Autodesk Fusion 360 part; units mm, degrees
(part 2 of 2)
sketch "Esquisse13" plane through (0, -12, 0) normal (0, -1, 0) x (1, 0, 0)
  line L0 (-488.8, 12) -> (-363.6, 12)
  line L1 (-363.6, 12) -> (-363.6, 0)
  line L2 (-363.6, 0) -> (-488.8, 0)
  line L3 (-488.8, 0) -> (-488.8, 12)
  line L4 (-238.4, 0) -> (-238.4, 12)
  line L5 (-238.4, 12) -> (-113.2, 12)
  line L6 (-113.2, 12) -> (-113.2, 0)
  line L7 (-113.2, 0) -> (-238.4, 0)
  circle A0 centre (-508.8, 6) radius 2
  circle A1 centre (-343.6, -186) radius 2
  circle A2 centre (-8, -186) radius 2
  circle A3 centre (-93.2, -186) radius 2
  circle A4 centre (-258.4, 6) radius 2
  circle A5 centre (-594, -186) radius 2
  circle A6 centre (-594, 6) radius 2
  circle A7 centre (-8, 6) radius 2
  circle A8 centre (-258.4, -186) radius 2
  circle A9 centre (-93.2, 6) radius 2
  circle A10 centre (-343.6, 6) radius 2
  circle A11 centre (-508.8, -186) radius 2
  line L8 (-363.6, -180) -> (-363.6, -192)
  line L9 (-363.6, -192) -> (-488.8, -192)
  line L10 (-488.8, -192) -> (-488.8, -180)
  line L11 (-488.8, -180) -> (-363.6, -180)
  line L12 (-238.4, -180) -> (-113.2, -180)
  line L13 (-113.2, -180) -> (-113.2, -192)
  line L14 (-113.2, -192) -> (-238.4, -192)
  line L15 (-238.4, -192) -> (-238.4, -180)
  line L16 (0, -332) -> (12, -332)
  line L17 (12, -332) -> (12, -241)
  line L18 (12, -241) -> (0, -241)
  line L19 (0, -241) -> (0, -150)
  line L20 (0, -150) -> (12, -150)
  line L21 (12, -150) -> (12, -59)
  line L22 (12, -59) -> (0, -59)
  line L23 (0, -59) -> (0, 32)
  line L24 (0, 32) -> (-602, 32)
  line L25 (-602, 32) -> (-602, -59)
  line L26 (-602, -59) -> (-614, -59)
  line L27 (-614, -59) -> (-614, -150)
  line L28 (-614, -150) -> (-602, -150)
  line L29 (-602, -150) -> (-602, -241)
  line L30 (-602, -241) -> (-614, -241)
  line L31 (-614, -241) -> (-614, -332)
  line L32 (-614, -332) -> (-602, -332)
  line L33 (-602, -332) -> (-602, -423)
  line L34 (-602, -423) -> (-614, -423)
  line L35 (-614, -423) -> (-614, -514)
  line L36 (-614, -514) -> (-602, -514)
  line L37 (-602, -514) -> (-602, -593)
  line L38 (-602, -593) -> (0, -593)
  line L39 (0, -593) -> (0, -514)
  line L40 (0, -514) -> (12, -514)
  line L41 (12, -514) -> (12, -423)
  line L42 (12, -423) -> (0, -423)
  line L43 (0, -423) -> (0, -332)
  line L44 (-602, 32) -> (0, 32)
  line L45 (0, 32) -> (0, -593)
  line L46 (0, -593) -> (-602, -593)
  line L47 (-602, -593) -> (-602, 32)
  line L48 (-20, -573) -> (-582, -573)
  line L49 (-582, -573) -> (-582, 12)
  line L50 (-582, 12) -> (-20, 12)
  line L51 (-20, 12) -> (-20, -573)
  line L52 (-582, -270.5) -> (-20, -270.5)
  line L53 (-20, -270.5) -> (-20, -290.5)
  line L54 (-20, -290.5) -> (-582, -290.5)
  line L55 (-582, -290.5) -> (-582, -270.5)
  dimension "d175" = 20
  dimension "d176" = 20
  constraint horizontal L44
  constraint vertical L45
  constraint horizontal L46
  constraint vertical L47
  constraint coincident L38.end L39.start
  constraint coincident L24.end L25.start
  constraint horizontal L52
  constraint vertical L53
  constraint horizontal L54
  constraint vertical L55
  constraint midpoint L51 L53
  constraint midpoint L49 L55
  measures "d176" distance of L52.end L53.end
extrude "Extrusion15" add sketch "Esquisse13" along normal blind 20 separate body contours L49 L51 L52 L53 L54 L55 | L19 L23 L24 L25 L29 L33 L37 L38 L39 L43 L44 L45 L46 L47 makes body 7
extrude "Extrusion16" cut sketch "Esquisse4" along normal blind 12 contours A12 L58 L76 | A12 L58 | A12 L76 bodies 3
sketch "Esquisse15" plane through (0, 0, 12) normal (0, 0, 1) x (1, 0, 0)
  line L0 (0, 845.1428) -> (0, 988)
  line L1 (0, 988) -> (-602, 988)
  line L2 (-602, 988) -> (-602, 845.1428)
  line L3 (-602, 845.1428) -> (-614, 845.1428)
  line L4 (-614, 845.1428) -> (-614, 702.2857)
  line L5 (-614, 702.2857) -> (-602, 702.2857)
  line L6 (-602, 702.2857) -> (-602, 559.4286)
  line L7 (-602, 559.4286) -> (-614, 559.4286)
  line L8 (-614, 559.4286) -> (-614, 416.5714)
  line L9 (-614, 416.5714) -> (-602, 416.5714)
  line L10 (-602, 416.5714) -> (-602, 273.7143)
  line L11 (-602, 273.7143) -> (-614, 273.7143)
  line L12 (-614, 273.7143) -> (-614, 130.8571)
  line L13 (-614, 130.8571) -> (-602, 130.8571)
  line L14 (-602, 130.8571) -> (-602, 0)
  line L15 (-602, 0) -> (-488.8, 0)
  line L16 (-488.8, 0) -> (-488.8, -12)
  line L17 (-488.8, -12) -> (-363.6, -12)
  line L18 (-363.6, -12) -> (-363.6, 0)
  line L19 (-363.6, 0) -> (-238.4, 0)
  line L20 (-238.4, 0) -> (-238.4, -12)
  line L21 (-238.4, -12) -> (-113.2, -12)
  line L22 (-113.2, -12) -> (-113.2, 0)
  line L23 (-113.2, 0) -> (0, 0)
  line L24 (0, 0) -> (0, 130.8571)
  line L25 (0, 130.8571) -> (12, 130.8571)
  line L26 (12, 130.8571) -> (12, 273.7143)
  line L27 (12, 273.7143) -> (0, 273.7143)
  line L28 (0, 273.7143) -> (0, 416.5714)
  line L29 (0, 416.5714) -> (12, 416.5714)
  line L30 (12, 416.5714) -> (12, 559.4286)
  line L31 (12, 559.4286) -> (0, 559.4286)
  line L32 (0, 559.4286) -> (0, 702.2857)
  line L33 (0, 702.2857) -> (12, 702.2857)
  line L34 (12, 702.2857) -> (12, 845.1428)
  line L35 (12, 845.1428) -> (0, 845.1428)
  line L36 (-301, 0) -> (-301, 988) construction
  circle A0 centre (-301, 40) radius 4
  circle A1 centre (-301, 390) radius 4
  circle A2 centre (-301, 740) radius 4
  dimension "d263" = 8
  dimension "d264" = 40
  dimension "d267" = 0
  dimension "d268" = 350
  constraint midpoint L19 L36.start
  constraint midpoint L1 L36.end
  constraint coincident L36 A0.centre
  measures "d263" diameter of A0
  measures "d264" distance of L36.start A0.centre
extrude "Extrusion17" cut sketch "Esquisse15" against normal blind 12 contours A0 | A1 | A2 bodies 5
copy_body "Corps->Comp1" bodies 1 removing the originals makes body 8 in component "Component"
copy_body "Corps->Comp2" bodies 6 removing the originals makes body 9 in component "Component'"
copy_body "Corps->Comp3" bodies 2 removing the originals makes body 10 in component "Component''"
copy_body "Corps->Comp4" bodies 4 removing the originals makes body 11 in component "Component'''"
copy_body "Corps->Comp5" bodies 5 removing the originals makes body 12 in component "Component''''"
copy_body "Corps->Comp6" bodies 3 removing the originals makes body 13 in component "Component'''''"
copy_body "Corps->Comp7" bodies 7 removing the originals makes body 14 in component "Component''''''"
sketch "Esquisse14" plane through (0, 0, 0) normal (0, 1, 0) x (1, 0, 0)
  line L0 (0, 0) -> (1250, 0)
  line L1 (1250, 0) -> (1250, -4000)
  line L2 (1250, -4000) -> (0, -4000)
  line L3 (0, -4000) -> (0, 0)
  line L4 (0, -4000) -> (-1250, -4000)
  line L5 (-1250, -4000) -> (-1250, 0)
  line L6 (-1250, 0) -> (0, 0)
  line L7 (0, 0) -> (0, -4000)
  line L8 (-1250, -4000) -> (-1650, -4000)
  line L9 (-1650, -4000) -> (-1650, 0)
  line L10 (-1650, 0) -> (-1250, 0)
  line L11 (-1250, 0) -> (-1250, -4000)
  dimension "d179" = 1250
  dimension "d180" = 4000
  dimension "d192" = 1250
  dimension "d193" = 400
  constraint horizontal L0
  constraint vertical L1
  constraint horizontal L2
  constraint vertical L3
  constraint coincident L0.start L3.end
  constraint horizontal L4
  constraint vertical L5
  constraint horizontal L6
  constraint vertical L7
  constraint horizontal L8
  constraint vertical L9
  constraint horizontal L10
  constraint vertical L11
  measures "d179" distance of L0.start L0.end
  measures "d180" distance of L0.start L2.end
  measures "d192" distance of L2.end L4.end
  measures "d193" distance of L9.end L5.end
other "Réorganiser1"
sketch "Esquisse1 (2)" plane through (0, 0, 0) normal (0, 1, 0) x (0, 0, -1) in component "Component'''''"
  circle A0 centre (-6, 508.8) radius 2
  circle A1 centre (186, 343.6) radius 2
  circle A2 centre (186, 8) radius 2
  circle A3 centre (186, 93.2) radius 2
  circle A4 centre (-6, 258.4) radius 2
  circle A5 centre (186, 594) radius 2
  circle A6 centre (-6, 594) radius 2
  circle A7 centre (-6, 8) radius 2
  circle A8 centre (186, 258.4) radius 2
  circle A9 centre (-6, 93.2) radius 2
  circle A10 centre (-6, 343.6) radius 2
  circle A11 centre (186, 508.8) radius 2
  line L0 (59, 602) -> (-32, 602)
  line L1 (-32, 290.802) -> (-32, 0)
  line L2 (-32, 0) -> (59, 0)
  line L3 (59, 0) -> (59, -12)
  line L4 (59, -12) -> (150, -12)
  line L5 (150, -12) -> (150, 0)
  line L6 (150, 0) -> (241, 0)
  line L7 (241, 0) -> (241, -12)
  line L8 (241, -12) -> (332, -12)
  line L9 (332, -12) -> (332, 0)
  line L10 (332, 0) -> (423, 0)
  line L11 (423, 0) -> (423, -12)
  line L12 (423, -12) -> (514, -12)
  line L13 (514, -12) -> (514, 0)
  line L14 (514, 0) -> (593, 0)
  line L15 (593, 0) -> (593, 602)
  line L16 (593, 602) -> (514, 602)
  line L17 (514, 602) -> (514, 614)
  line L18 (514, 614) -> (423, 614)
  line L19 (423, 614) -> (423, 602)
  line L20 (423, 602) -> (332, 602)
  line L21 (332, 602) -> (332, 614)
  line L22 (332, 614) -> (241, 614)
  line L23 (241, 614) -> (241, 602)
  line L24 (241, 602) -> (150, 602)
  line L25 (150, 602) -> (150, 614)
  line L26 (150, 614) -> (59, 614)
  line L27 (59, 614) -> (59, 602)
  line L28 (-12, 488.8) -> (0, 488.8)
  line L29 (0, 488.8) -> (0, 363.6)
  line L30 (0, 363.6) -> (-12, 363.6)
  line L31 (-12, 363.6) -> (-12, 488.8)
  line L32 (180, 488.8) -> (192, 488.8)
  line L33 (192, 488.8) -> (192, 363.6)
  line L34 (192, 363.6) -> (180, 363.6)
  line L35 (180, 363.6) -> (180, 488.8)
  line L36 (180, 238.4) -> (192, 238.4)
  line L37 (192, 238.4) -> (192, 113.2)
  line L38 (192, 113.2) -> (180, 113.2)
  line L39 (180, 113.2) -> (180, 238.4)
  line L40 (-12, 238.4) -> (0, 238.4)
  line L41 (0, 238.4) -> (0, 113.2)
  line L42 (0, 113.2) -> (-12, 113.2)
  line L43 (-12, 113.2) -> (-12, 238.4)
  arc A12 (-32, 290.802) -> (-32, 311.198) centre (-24.6, 301) ccw
  line L44 (-32, 602) -> (-32, 311.198)
  point P0 (-9.6665, 115.5335)
  point P1 (-9.6665, 236.0665)
  point P2 (-2.3335, 236.0665)
  point P3 (-2.3335, 115.5335)
  point P4 (-2.3335, 486.4665)
  point P5 (-2.3335, 365.9335)
  point P6 (-9.6665, 486.4665)
  point P7 (-9.6665, 365.9335)
  point P8 (182.3335, 115.5335)
  point P9 (182.3335, 236.0665)
  point P10 (189.6665, 236.0665)
  point P11 (189.6665, 115.5335)
  point P12 (189.6665, 486.4665)
  point P13 (189.6665, 365.9335)
  point P14 (182.3335, 486.4665)
  point P15 (182.3335, 365.9335)
  point P16 (56.6665, 604.3335)
  point P17 (152.3335, 604.3335)
  point P18 (238.6665, 604.3335)
  point P19 (334.3335, 604.3335)
  point P20 (420.6665, 604.3335)
  point P21 (516.3335, 604.3335)
  point P22 (56.6665, -2.3335)
  point P23 (152.3335, -2.3335)
  point P24 (238.6665, -2.3335)
  point P25 (334.3335, -2.3335)
  point P26 (420.6665, -2.3335)
  point P27 (516.3335, -2.3335)
hole "Perçage1" at (-115.5335, 0, 9.6665) at (-236.0665, 0, 9.6665) at (-236.0665, 0, 2.3335) at (-115.5335, 0, 2.3335) at (-486.4665, 0, 2.3335) at (-365.9335, 0, 2.3335) at (-486.4665, 0, 9.6665) at (-365.9335, 0, 9.6665) at (-115.5335, 0, -182.3335) at (-236.0665, 0, -182.3335) at (-236.0665, 0, -189.6665) at (-115.5335, 0, -189.6665) at (-486.4665, 0, -189.6665) at (-365.9335, 0, -189.6665) at (-486.4665, 0, -182.3335) at (-365.9335, 0, -182.3335) direction (0, -1, 0) diameter 6 depth 12 tip angle 180 bodies 13 in component "Component'''''"
hole "Perçage2" at (-604.3335, 0, -56.6665) at (-604.3335, 0, -152.3335) at (-604.3335, 0, -238.6665) at (-604.3335, 0, -334.3335) at (-604.3335, 0, -420.6665) at (-604.3335, 0, -516.3335) at (2.3335, 0, -56.6665) at (2.3335, 0, -152.3335) at (2.3335, 0, -238.6665) at (2.3335, 0, -334.3335) at (2.3335, 0, -420.6665) at (2.3335, 0, -516.3335) direction (0, -1, 0) diameter 6 depth 12 tip angle 180 bodies 13 in component "Component'''''"
sketch "Esquisse1 (3)" plane through (0, 0, -605) normal (0, 0, -1) x (-1, 0, 0) in component "Component'"
  spline S0 degree 3 poles (527.6621, 131.6413) (528.5608, 136.7718) (530.453, 141.6777) (536.0113, 150.4881) (539.6243, 154.3083) (547.2342, 159.7245) (550.9515, 161.5844) (558.8233, 164.0997) (562.9304, 164.7399) (567.0623, 164.7399) knots 0 0 0 0 1.562578 1.562578 3.125156 3.125156 4.364729 4.364729 5.604303 5.604303 5.604303 5.604303
  spline S1 degree 5 poles (527.6621, 131.6413) (526.9913, 127.8114) (525.3201, 119.0874) (522.2246, 106.0357) (516.6629, 89.886) (506.2841, 73.0853) (490.6132, 60.2852) (469.9401, 52.3455) (445.0295, 48.3011) (417.063, 46.7974) (393.2682, 46.4893) (375.0825, 46.2548) (362.8686, 46.0302) (356.739, 45.9008) knots 0.124254 0.124254 0.124254 0.124254 0.124254 0.124254 0.2 0.3 0.4 0.5 0.6 0.7 0.8 0.9 1 1 1 1 1 1
  line L0 (356.739, 45.9008) -> (245.261, 45.9008)
  spline S2 degree 5 poles (245.261, 45.9008) (239.1314, 46.0302) (226.9175, 46.2548) (208.7318, 46.4893) (184.937, 46.7974) (156.9705, 48.3011) (132.0599, 52.3455) (111.3868, 60.2852) (95.7159, 73.0853) (85.3371, 89.886) (79.7754, 106.0357) (76.6799, 119.0874) (75.0087, 127.8114) (74.3379, 131.6413) knots -1 -1 -1 -1 -1 -1 -0.9 -0.8 -0.7 -0.6 -0.5 -0.4 -0.3 -0.2 -0.124254 -0.124254 -0.124254 -0.124254 -0.124254 -0.124254
  spline S3 degree 3 poles (34.9377, 164.7399) (40.1463, 164.7399) (45.3051, 163.7226) (54.9424, 159.7677) (59.3287, 156.8679) (65.9766, 150.3067) (68.45, 146.966) (72.2857, 139.6463) (73.625, 135.7113) (74.3379, 131.6413) knots 0 0 0 0 1.562578 1.562578 3.125156 3.125156 4.364729 4.364729 5.604303 5.604303 5.604303 5.604303
  line L1 (34.9377, 164.7399) -> (-6, 164.7399)
  line L2 (-6, 164.7399) -> (-6, 158.7399)
  line L3 (-6, 158.7399) -> (0, 158.7399)
  line L4 (0, 158.7399) -> (0, -44.13)
  line L5 (0, -44.13) -> (-12, -44.13)
  line L6 (-12, -44.13) -> (-12, -56.13)
  line L7 (-12, -56.13) -> (614, -56.13)
  line L8 (614, -56.13) -> (614, -44.13)
  line L9 (614, -44.13) -> (602, -44.13)
  line L10 (602, -44.13) -> (602, 158.7399)
  line L11 (602, 158.7399) -> (608, 158.7399)
  line L12 (608, 158.7399) -> (608, 164.7399)
  line L13 (608, 164.7399) -> (567.0623, 164.7399)
  point P0 (604.3335, 156.4065)
  point P1 (-2.3335, 156.4065)
  point P2 (-2.3335, -41.7966)
  point P3 (604.3335, -41.7966)
hole "Perçage1'" at (-604.3335, 156.4065, -605) at (2.3335, 156.4065, -605) direction (0, 0, 1) diameter 6 depth 6 tip angle 180 bodies 9 in component "Component'"
hole "Perçage2'" at (2.3335, -41.7966, -605) at (-604.3335, -41.7966, -605) direction (0, 0, 1) diameter 6 depth 12 tip angle 180 bodies 9 in component "Component'"
sketch "Esquisse1 (4)" plane through (0, 0, 12) normal (0, 0, 1) x (0, 1, 0) in component "Component''''"
  line L0 (845.1428, 0) -> (988, 0)
  line L1 (988, 0) -> (988, 602)
  line L2 (988, 602) -> (845.1428, 602)
  line L3 (845.1428, 602) -> (845.1428, 614)
  line L4 (845.1428, 614) -> (702.2857, 614)
  line L5 (702.2857, 614) -> (702.2857, 602)
  line L6 (702.2857, 602) -> (559.4286, 602)
  line L7 (559.4286, 602) -> (559.4286, 614)
  line L8 (559.4286, 614) -> (416.5714, 614)
  line L9 (416.5714, 614) -> (416.5714, 602)
  line L10 (416.5714, 602) -> (273.7143, 602)
  line L11 (273.7143, 602) -> (273.7143, 614)
  line L12 (273.7143, 614) -> (130.8571, 614)
  line L13 (130.8571, 614) -> (130.8571, 602)
  line L14 (130.8571, 602) -> (0, 602)
  line L15 (0, 602) -> (0, 488.8)
  line L16 (0, 488.8) -> (-12, 488.8)
  line L17 (-12, 488.8) -> (-12, 363.6)
  line L18 (-12, 363.6) -> (0, 363.6)
  line L19 (0, 363.6) -> (0, 238.4)
  line L20 (0, 238.4) -> (-12, 238.4)
  line L21 (-12, 238.4) -> (-12, 113.2)
  line L22 (-12, 113.2) -> (0, 113.2)
  line L23 (0, 113.2) -> (0, 0)
  line L24 (0, 0) -> (130.8571, 0)
  line L25 (130.8571, 0) -> (130.8571, -12)
  line L26 (130.8571, -12) -> (273.7143, -12)
  line L27 (273.7143, -12) -> (273.7143, 0)
  line L28 (273.7143, 0) -> (416.5714, 0)
  line L29 (416.5714, 0) -> (416.5714, -12)
  line L30 (416.5714, -12) -> (559.4286, -12)
  line L31 (559.4286, -12) -> (559.4286, 0)
  line L32 (559.4286, 0) -> (702.2857, 0)
  line L33 (702.2857, 0) -> (702.2857, -12)
  line L34 (702.2857, -12) -> (845.1428, -12)
  line L35 (845.1428, -12) -> (845.1428, 0)
  circle A0 centre (40, 301) radius 4
  circle A1 centre (390, 301) radius 4
  circle A2 centre (740, 301) radius 4
  point P0 (-2.3335, 491.1335)
  point P1 (-2.3335, 361.2665)
  point P2 (-2.3335, 240.7335)
  point P3 (-2.3335, 110.8665)
  point P4 (128.5237, 604.3335)
  point P5 (276.0477, 604.3335)
  point P6 (414.238, 604.3335)
  point P7 (699.9523, 604.3335)
  point P8 (847.4763, 604.3335)
  point P9 (561.762, 604.3335)
  point P10 (414.238, -2.3335)
  point P11 (561.762, -2.3335)
  point P12 (276.0477, -2.3335)
  point P13 (699.9523, -2.3335)
  point P14 (128.5237, -2.3335)
  point P15 (847.4763, -2.3335)
hole "Perçage1''" at (-491.1335, -2.3335, 12) at (-361.2665, -2.3335, 12) at (-240.7335, -2.3335, 12) at (-110.8665, -2.3335, 12) direction (0, 0, -1) diameter 6 depth 12 tip angle 180 bodies 12 in component "Component''''"
hole "Perçage2''" at (-604.3335, 276.0477, 12) at (-604.3335, 414.238, 12) at (-604.3335, 699.9523, 12) at (-604.3335, 847.4763, 12) at (-604.3335, 561.762, 12) at (2.3335, 414.238, 12) at (2.3335, 561.762, 12) at (2.3335, 276.0477, 12) at (2.3335, 699.9523, 12) at (2.3335, 128.5237, 12) at (2.3335, 847.4763, 12) direction (0, 0, -1) diameter 6 depth 12 tip angle 180 bodies 12 in component "Component''''"
hole "Perçage3" at (-604.3335, 128.5237, 12) direction (0, 0, -1) diameter 6 depth 12 tip angle 180 bodies 12 in component "Component''''"
sketch "Esquisse1 (5)" plane through (0, 0, 0) normal (-1, 0, 0) x (0, 0, 1) in component "Component"
  arc A0 (32.1287, 968) -> (12.1287, 988) centre (12.1287, 968) ccw
  line L0 (12.1287, 988) -> (-209.8465, 988)
  arc A1 (-209.8465, 988) -> (-227.5983, 977.2127) centre (-209.8465, 968) ccw
  line L1 (-227.5983, 977.2127) -> (-569.8721, 317.6877)
  arc A2 (-569.8721, 317.6877) -> (-605, 173.7399) centre (-292.5, 173.7399) ccw
  line L2 (-605, 173.7399) -> (-593, 173.7399)
  line L3 (-593, 173.7399) -> (-593, 158.7399)
  line L4 (-593, 158.7399) -> (-593, 150.7399)
  line L5 (-593, 150.7399) -> (-599, 150.7399)
  line L6 (-599, 150.7399) -> (-599, 158.7399)
  line L7 (-599, 158.7399) -> (-605, 158.7399)
  line L8 (-605, 158.7399) -> (-605, 16.37)
  line L9 (-605, 16.37) -> (-626.1765, -28.9242)
  arc A3 (-626.1765, -28.9242) -> (-585.3674, -68.3537) centre (-599, -41.63) ccw
  line L10 (-585.3674, -68.3537) -> (-514.1044, -32)
  line L11 (-514.1044, -32) -> (12, -32)
  arc A4 (12, -32) -> (32, -12) centre (12, -12) ccw
  line L12 (32, -12) -> (32.1287, -12)
  line L13 (32.1287, -12) -> (32.1287, 968)
  line L14 (-59, 0) -> (-59, -12)
  line L15 (-59, -12) -> (-150, -12)
  line L16 (-150, -12) -> (-150, 0)
  line L17 (-150, 0) -> (-59, 0)
  line L18 (-192, 273.7143) -> (-180, 273.7143)
  line L19 (-180, 273.7143) -> (-180, 130.8571)
  line L20 (-180, 130.8571) -> (-192, 130.8571)
  line L21 (-192, 130.8571) -> (-192, 273.7143)
  line L22 (-180, 559.4286) -> (-180, 416.5714)
  line L23 (-180, 416.5714) -> (-192, 416.5714)
  line L24 (-192, 416.5714) -> (-192, 559.4286)
  line L25 (-192, 559.4286) -> (-180, 559.4286)
  line L26 (0, 702.2857) -> (0, 845.1428)
  line L27 (0, 845.1428) -> (12, 845.1428)
  line L28 (12, 845.1428) -> (12, 702.2857)
  line L29 (12, 702.2857) -> (0, 702.2857)
  line L30 (-241, 0) -> (-241, -12)
  line L31 (-241, -12) -> (-332, -12)
  line L32 (-332, -12) -> (-332, 0)
  line L33 (-332, 0) -> (-241, 0)
  line L34 (0, 130.8571) -> (0, 273.7143)
  line L35 (0, 273.7143) -> (12, 273.7143)
  line L36 (12, 273.7143) -> (12, 130.8571)
  line L37 (12, 130.8571) -> (0, 130.8571)
  line L38 (-180, 845.1428) -> (-180, 702.2857)
  line L39 (-180, 702.2857) -> (-192, 702.2857)
  line L40 (-192, 702.2857) -> (-192, 845.1428)
  line L41 (-192, 845.1428) -> (-180, 845.1428)
  line L42 (0, 416.5714) -> (0, 559.4286)
  line L43 (0, 559.4286) -> (12, 559.4286)
  line L44 (12, 559.4286) -> (12, 416.5714)
  line L45 (12, 416.5714) -> (0, 416.5714)
  line L46 (-423, 0) -> (-423, -12)
  line L47 (-423, -12) -> (-514, -12)
  line L48 (-514, -12) -> (-514, 0)
  line L49 (-514, 0) -> (-423, 0)
  line L50 (-593, -27.13) -> (-593, -35.13)
  arc A5 (-593, -48.13) -> (-593, -35.13) centre (-599, -41.63) ccw
  line L51 (-593, -48.13) -> (-593, -56.13)
  line L52 (-593, -56.13) -> (-605, -56.13)
  line L53 (-605, -56.13) -> (-605, -48.13)
  arc A6 (-605, -35.13) -> (-605, -48.13) centre (-599, -41.63) ccw
  line L54 (-605, -35.13) -> (-605, -27.13)
  line L55 (-605, -27.13) -> (-593, -27.13)
  circle A7 centre (6, 115.8571) radius 2
  circle A8 centre (-161.8713, -6) radius 2
  circle A9 centre (6, 288.7143) radius 2
  circle A10 centre (6, 401.5714) radius 2
  circle A11 centre (-229, -6) radius 2
  circle A12 centre (-343.8713, -6) radius 2
  circle A13 centre (6, 574.4286) radius 2
  circle A14 centre (6, 687.2857) radius 2
  circle A15 centre (6, 860.1428) radius 2
  circle A16 centre (-525.8713, -6) radius 2
  circle A17 centre (-581, -6) radius 2
  circle A18 centre (-186, 687.2857) radius 2
  circle A19 centre (-411, -6) radius 2
  circle A20 centre (6, 15) radius 2
  circle A21 centre (6, 973) radius 2
  circle A22 centre (-186, 288.7143) radius 2
  circle A23 centre (-186, 860.1428) radius 2
  circle A24 centre (-186, 973) radius 2
  circle A25 centre (-186, 401.5714) radius 2
  circle A26 centre (-186, 574.4286) radius 2
  circle A27 centre (-186, 15) radius 2
  circle A28 centre (-186, 115.8571) radius 2
  circle A29 centre (20.1287, -6) radius 2
  circle A30 centre (-47, -6) radius 2
  point P0 (-61.3335, -2.3335)
  point P1 (-61.3335, -9.6665)
  point P2 (-147.6665, -2.3335)
  point P3 (-147.6665, -9.6665)
  point P4 (-189.6665, 271.3808)
  point P5 (-182.3335, 271.3808)
  point P6 (-189.6665, 133.1906)
  point P7 (-182.3335, 133.1906)
  point P8 (-182.3335, 557.0951)
  point P9 (-182.3335, 418.9049)
  point P10 (-189.6665, 557.0951)
  point P11 (-189.6665, 418.9049)
  point P12 (2.3335, 704.6192)
  point P13 (2.3335, 842.8094)
  point P14 (9.6665, 704.6192)
  point P15 (9.6665, 842.8094)
  point P16 (-243.3335, -2.3335)
  point P17 (-243.3335, -9.6665)
  point P18 (-329.6665, -2.3335)
  point P19 (-329.6665, -9.6665)
  point P20 (2.3335, 133.1906)
  point P21 (2.3335, 271.3808)
  point P22 (9.6665, 133.1906)
  point P23 (9.6665, 271.3808)
  point P24 (-182.3335, 842.8094)
  point P25 (-182.3335, 704.6192)
  point P26 (-189.6665, 842.8094)
  point P27 (-189.6665, 704.6192)
  point P28 (2.3335, 418.9049)
  point P29 (2.3335, 557.0951)
  point P30 (9.6665, 418.9049)
  point P31 (9.6665, 557.0951)
  point P32 (-425.3335, -2.3335)
  point P33 (-425.3335, -9.6665)
  point P34 (-511.6665, -2.3335)
  point P35 (-511.6665, -9.6665)
  point P36 (-595.3335, -29.4635)
  point P37 (-602.6665, -29.4635)
  point P38 (-595.3335, -53.7966)
  point P39 (-602.6665, -53.7966)
  point P40 (-608.2214, 17.0858)
  point P41 (-513.3333, -35.2086)
  point P42 (-595.3335, 153.0734)
  point P43 (-596.6665, 153.0734)
  point P44 (-595.3335, 171.4065)
hole "Perçage1'''" at (0, 153.0734, -595.3335) at (0, 153.0734, -596.6665) at (0, 171.4065, -595.3335) direction (1, 0, 0) diameter 6 depth 6 tip angle 180 bodies 8 in component "Component"
hole "Perçage2'''" at (0, -2.3335, -61.3335) at (0, -9.6665, -61.3335) at (0, -2.3335, -147.6665) at (0, -9.6665, -147.6665) at (0, 271.3808, -189.6665) at (0, 271.3808, -182.3335) at (0, 133.1906, -189.6665) at (0, 133.1906, -182.3335) at (0, 557.0951, -182.3335) at (0, 418.9049, -182.3335) at (0, 557.0951, -189.6665) at (0, 418.9049, -189.6665) at (0, 704.6192, 2.3335) at (0, 842.8094, 2.3335) at (0, 704.6192, 9.6665) at (0, 842.8094, 9.6665) at (0, -2.3335, -243.3335) at (0, -9.6665, -243.3335) at (0, -2.3335, -329.6665) at (0, -9.6665, -329.6665) at (0, 133.1906, 2.3335) at (0, 271.3808, 2.3335) at (0, 133.1906, 9.6665) at (0, 271.3808, 9.6665) at (0, 842.8094, -182.3335) at (0, 704.6192, -182.3335) at (0, 842.8094, -189.6665) at (0, 704.6192, -189.6665) at (0, 418.9049, 2.3335) at (0, 557.0951, 2.3335) at (0, 418.9049, 9.6665) at (0, 557.0951, 9.6665) at (0, -2.3335, -425.3335) at (0, -9.6665, -425.3335) at (0, -2.3335, -511.6665) at (0, -9.6665, -511.6665) at (0, -29.4635, -595.3335) at (0, -29.4635, -602.6665) at (0, -53.7966, -595.3335) at (0, -53.7966, -602.6665) at (0, 17.0858, -608.2214) at (0, -35.2086, -513.3333) direction (1, 0, 0) diameter 6 depth 12 tip angle 180 bodies 8 in component "Component"
sketch "Esquisse1 (6)" plane through (-602, 0, 0) normal (1, 0, 0) x (0, 0, 1) in component "Component''"
  arc A0 (12.1287, -988) -> (32.1287, -968) centre (12.1287, -968) ccw
  line L0 (32.1287, -968) -> (32.1287, 12)
  line L1 (32.1287, 12) -> (32, 12)
  arc A1 (32, 12) -> (12, 32) centre (12, 12) ccw
  line L2 (12, 32) -> (-514.1044, 32)
  line L3 (-514.1044, 32) -> (-585.3674, 68.3537)
  arc A2 (-585.3674, 68.3537) -> (-626.1765, 28.9242) centre (-599, 41.63) ccw
  line L4 (-626.1765, 28.9242) -> (-605, -16.37)
  line L5 (-605, -16.37) -> (-605, -158.7399)
  line L6 (-605, -158.7399) -> (-599, -158.7399)
  line L7 (-599, -158.7399) -> (-599, -150.7399)
  line L8 (-599, -150.7399) -> (-593, -150.7399)
  line L9 (-593, -150.7399) -> (-593, -158.7399)
  line L10 (-593, -158.7399) -> (-593, -173.7399)
  line L11 (-593, -173.7399) -> (-605, -173.7399)
  arc A3 (-605, -173.7399) -> (-569.8721, -317.6877) centre (-292.5, -173.7399) ccw
  line L12 (-569.8721, -317.6877) -> (-227.5983, -977.2127)
  arc A4 (-227.5983, -977.2127) -> (-209.8465, -988) centre (-209.8465, -968) ccw
  line L13 (-209.8465, -988) -> (12.1287, -988)
  line L14 (-59, 12) -> (-59, 0)
  line L15 (-59, 0) -> (-150, 0)
  line L16 (-150, 0) -> (-150, 12)
  line L17 (-150, 12) -> (-59, 12)
  line L18 (-180, -273.7143) -> (-192, -273.7143)
  line L19 (-192, -273.7143) -> (-192, -130.8571)
  line L20 (-192, -130.8571) -> (-180, -130.8571)
  line L21 (-180, -130.8571) -> (-180, -273.7143)
  line L22 (-180, -416.5714) -> (-180, -559.4286)
  line L23 (-180, -559.4286) -> (-192, -559.4286)
  line L24 (-192, -559.4286) -> (-192, -416.5714)
  line L25 (-192, -416.5714) -> (-180, -416.5714)
  line L26 (0, -845.1428) -> (0, -702.2857)
  line L27 (0, -702.2857) -> (12, -702.2857)
  line L28 (12, -702.2857) -> (12, -845.1428)
  line L29 (12, -845.1428) -> (0, -845.1428)
  line L30 (-241, 12) -> (-241, 0)
  line L31 (-241, 0) -> (-332, 0)
  line L32 (-332, 0) -> (-332, 12)
  line L33 (-332, 12) -> (-241, 12)
  line L34 (0, -273.7143) -> (0, -130.8571)
  line L35 (0, -130.8571) -> (12, -130.8571)
  line L36 (12, -130.8571) -> (12, -273.7143)
  line L37 (12, -273.7143) -> (0, -273.7143)
  line L38 (-180, -702.2857) -> (-180, -845.1428)
  line L39 (-180, -845.1428) -> (-192, -845.1428)
  line L40 (-192, -845.1428) -> (-192, -702.2857)
  line L41 (-192, -702.2857) -> (-180, -702.2857)
  line L42 (0, -559.4286) -> (0, -416.5714)
  line L43 (0, -416.5714) -> (12, -416.5714)
  line L44 (12, -416.5714) -> (12, -559.4286)
  line L45 (12, -559.4286) -> (0, -559.4286)
  line L46 (-423, 12) -> (-423, 0)
  line L47 (-423, 0) -> (-514, 0)
  line L48 (-514, 0) -> (-514, 12)
  line L49 (-514, 12) -> (-423, 12)
  line L50 (-593, 35.13) -> (-593, 27.13)
  line L51 (-593, 27.13) -> (-605, 27.13)
  line L52 (-605, 27.13) -> (-605, 35.13)
  arc A5 (-605, 48.13) -> (-605, 35.13) centre (-599, 41.63) ccw
  line L53 (-605, 48.13) -> (-605, 56.13)
  line L54 (-605, 56.13) -> (-593, 56.13)
  line L55 (-593, 56.13) -> (-593, 48.13)
  arc A6 (-593, 35.13) -> (-593, 48.13) centre (-599, 41.63) ccw
  circle A7 centre (6, -115.8571) radius 2
  circle A8 centre (-161.8713, 6) radius 2
  circle A9 centre (6, -288.7143) radius 2
  circle A10 centre (6, -401.5714) radius 2
  circle A11 centre (-229, 6) radius 2
  circle A12 centre (-343.8713, 6) radius 2
  circle A13 centre (6, -574.4286) radius 2
  circle A14 centre (6, -687.2857) radius 2
  circle A15 centre (6, -860.1428) radius 2
  circle A16 centre (-525.8713, 6) radius 2
  circle A17 centre (-581, 6) radius 2
  circle A18 centre (-186, -687.2857) radius 2
  circle A19 centre (-411, 6) radius 2
  circle A20 centre (6, -15) radius 2
  circle A21 centre (6, -973) radius 2
  circle A22 centre (-186, -288.7143) radius 2
  circle A23 centre (-186, -860.1428) radius 2
  circle A24 centre (-186, -973) radius 2
  circle A25 centre (-186, -401.5714) radius 2
  circle A26 centre (-186, -574.4286) radius 2
  circle A27 centre (-186, -15) radius 2
  circle A28 centre (-186, -115.8571) radius 2
  circle A29 centre (20.1287, 6) radius 2
  circle A30 centre (-47, 6) radius 2
  point P0 (-513.3333, 35.2086)
  point P1 (-61.3335, 9.6665)
  point P2 (-61.3335, 2.3335)
  point P3 (-147.6665, 2.3335)
  point P4 (-147.6665, 9.6665)
  point P5 (-182.3335, -271.3808)
  point P6 (-189.6665, -271.3808)
  point P7 (-189.6665, -133.1906)
  point P8 (-182.3335, -133.1906)
  point P9 (-182.3335, -418.9049)
  point P10 (-182.3335, -557.0951)
  point P11 (-189.6665, -557.0951)
  point P12 (-189.6665, -418.9049)
  point P13 (2.3335, -842.8094)
  point P14 (2.3335, -704.6192)
  point P15 (9.6665, -704.6192)
  point P16 (9.6665, -842.8094)
  point P17 (-243.3335, 9.6665)
  point P18 (-243.3335, 2.3335)
  point P19 (-329.6665, 2.3335)
  point P20 (-329.6665, 9.6665)
  point P21 (2.3335, -271.3808)
  point P22 (2.3335, -133.1906)
  point P23 (9.6665, -133.1906)
  point P24 (9.6665, -271.3808)
  point P25 (-182.3335, -704.6192)
  point P26 (-182.3335, -842.8094)
  point P27 (-189.6665, -842.8094)
  point P28 (-189.6665, -704.6192)
  point P29 (2.3335, -557.0951)
  point P30 (2.3335, -418.9049)
  point P31 (9.6665, -418.9049)
  point P32 (9.6665, -557.0951)
  point P33 (-425.3335, 9.6665)
  point P34 (-425.3335, 2.3335)
  point P35 (-511.6665, 2.3335)
  point P36 (-511.6665, 9.6665)
  point P37 (-595.3335, 29.4635)
  point P38 (-602.6665, 29.4635)
  point P39 (-595.3335, 53.7966)
  point P40 (-602.6665, 53.7966)
  point P41 (-608.2214, -17.0858)
  point P42 (-595.3335, -153.0734)
  point P43 (-596.6665, -153.0734)
  point P44 (-595.3335, -171.4065)
hole "Perçage1''''" at (-602, 153.0734, -595.3335) at (-602, 153.0734, -596.6665) at (-602, 171.4065, -595.3335) direction (-1, 0, 0) diameter 6 depth 6 tip angle 180 bodies 10 in component "Component''"
hole "Perçage2''''" at (-602, -35.2086, -513.3333) at (-602, -9.6665, -61.3335) at (-602, -2.3335, -61.3335) at (-602, -2.3335, -147.6665) at (-602, -9.6665, -147.6665) at (-602, 271.3808, -182.3335) at (-602, 271.3808, -189.6665) at (-602, 133.1906, -189.6665) at (-602, 133.1906, -182.3335) at (-602, 418.9049, -182.3335) at (-602, 557.0951, -182.3335) at (-602, 557.0951, -189.6665) at (-602, 418.9049, -189.6665) at (-602, 842.8094, 2.3335) at (-602, 704.6192, 2.3335) at (-602, 704.6192, 9.6665) at (-602, 842.8094, 9.6665) at (-602, -9.6665, -243.3335) at (-602, -2.3335, -243.3335) at (-602, -2.3335, -329.6665) at (-602, -9.6665, -329.6665) at (-602, 271.3808, 2.3335) at (-602, 133.1906, 2.3335) at (-602, 133.1906, 9.6665) at (-602, 271.3808, 9.6665) at (-602, 704.6192, -182.3335) at (-602, 842.8094, -182.3335) at (-602, 842.8094, -189.6665) at (-602, 704.6192, -189.6665) at (-602, 557.0951, 2.3335) at (-602, 418.9049, 2.3335) at (-602, 418.9049, 9.6665) at (-602, 557.0951, 9.6665) at (-602, -9.6665, -425.3335) at (-602, -2.3335, -425.3335) at (-602, -2.3335, -511.6665) at (-602, -9.6665, -511.6665) at (-602, -29.4635, -595.3335) at (-602, -29.4635, -602.6665) at (-602, -53.7966, -595.3335) at (-602, -53.7966, -602.6665) at (-602, 17.0858, -608.2214) direction (-1, 0, 0) diameter 6 depth 12 tip angle 180 bodies 10 in component "Component''"
sketch "Esquisse2 (2)" plane through (0, 0, 12) normal (0, 0, 1) x (0, 1, 0) in component "Component''''"
  arc A0 (126.6382, 602) -> (130.4092, 602) centre (128.5237, 604.3335) ccw
  line L0 (126.6382, 602) -> (0, 602)
  line L1 (0, 602) -> (0, 493.0189)
  arc A1 (0, 489.248) -> (0, 493.0189) centre (-2.3335, 491.1335) ccw
  line L2 (0, 489.248) -> (0, 488.8)
  line L3 (0, 488.8) -> (-0.448, 488.8)
  arc A2 (-4.2189, 488.8) -> (-0.448, 488.8) centre (-2.3335, 491.1335) ccw
  line L4 (-4.2189, 488.8) -> (-12, 488.8)
  line L5 (-12, 488.8) -> (-12, 363.6)
  line L6 (-12, 363.6) -> (-4.2189, 363.6)
  arc A3 (-0.448, 363.6) -> (-4.2189, 363.6) centre (-2.3335, 361.2665) ccw
  line L7 (-0.448, 363.6) -> (0, 363.6)
  line L8 (0, 363.6) -> (0, 363.152)
  arc A4 (0, 359.3811) -> (0, 363.152) centre (-2.3335, 361.2665) ccw
  line L9 (0, 359.3811) -> (0, 242.6189)
  arc A5 (0, 238.848) -> (0, 242.6189) centre (-2.3335, 240.7335) ccw
  line L10 (0, 238.848) -> (0, 238.4)
  line L11 (0, 238.4) -> (-0.448, 238.4)
  arc A6 (-4.2189, 238.4) -> (-0.448, 238.4) centre (-2.3335, 240.7335) ccw
  line L12 (-4.2189, 238.4) -> (-12, 238.4)
  line L13 (-12, 238.4) -> (-12, 113.2)
  line L14 (-12, 113.2) -> (-4.2189, 113.2)
  arc A7 (-0.448, 113.2) -> (-4.2189, 113.2) centre (-2.3335, 110.8665) ccw
  line L15 (-0.448, 113.2) -> (0, 113.2)
  line L16 (0, 113.2) -> (0, 112.752)
  arc A8 (0, 108.9811) -> (0, 112.752) centre (-2.3335, 110.8665) ccw
  line L17 (0, 108.9811) -> (0, 0)
  line L18 (0, 0) -> (126.6382, 0)
  arc A9 (130.4092, 0) -> (126.6382, 0) centre (128.5237, -2.3335) ccw
  line L19 (130.4092, 0) -> (130.8571, 0)
  line L20 (130.8571, 0) -> (130.8571, -0.448)
  arc A10 (130.8571, -4.2189) -> (130.8571, -0.448) centre (128.5237, -2.3335) ccw
  line L21 (130.8571, -4.2189) -> (130.8571, -12)
  line L22 (130.8571, -12) -> (273.7143, -12)
  line L23 (273.7143, -12) -> (273.7143, -4.2189)
  arc A11 (273.7143, -0.448) -> (273.7143, -4.2189) centre (276.0477, -2.3335) ccw
  line L24 (273.7143, -0.448) -> (273.7143, 0)
  line L25 (273.7143, 0) -> (274.1623, 0)
  arc A12 (277.9332, 0) -> (274.1623, 0) centre (276.0477, -2.3335) ccw
  line L26 (277.9332, 0) -> (412.3525, 0)
  arc A13 (416.1234, 0) -> (412.3525, 0) centre (414.238, -2.3335) ccw
  line L27 (416.1234, 0) -> (416.5714, 0)
  line L28 (416.5714, 0) -> (416.5714, -0.448)
  arc A14 (416.5714, -4.2189) -> (416.5714, -0.448) centre (414.238, -2.3335) ccw
  line L29 (416.5714, -4.2189) -> (416.5714, -12)
  line L30 (416.5714, -12) -> (559.4286, -12)
  line L31 (559.4286, -12) -> (559.4286, -4.2189)
  arc A15 (559.4286, -0.448) -> (559.4286, -4.2189) centre (561.762, -2.3335) ccw
  line L32 (559.4286, -0.448) -> (559.4286, 0)
  line L33 (559.4286, 0) -> (559.8765, 0)
  arc A16 (563.6475, 0) -> (559.8765, 0) centre (561.762, -2.3335) ccw
  line L34 (563.6475, 0) -> (698.0668, 0)
  arc A17 (701.8377, 0) -> (698.0668, 0) centre (699.9523, -2.3335) ccw
  line L35 (701.8377, 0) -> (702.2857, 0)
  line L36 (702.2857, 0) -> (702.2857, -0.448)
  arc A18 (702.2857, -4.2189) -> (702.2857, -0.448) centre (699.9523, -2.3335) ccw
  line L37 (702.2857, -4.2189) -> (702.2857, -12)
  line L38 (702.2857, -12) -> (845.1428, -12)
  line L39 (845.1428, -12) -> (845.1428, -4.2189)
  arc A19 (845.1428, -0.448) -> (845.1428, -4.2189) centre (847.4763, -2.3335) ccw
  line L40 (845.1428, -0.448) -> (845.1428, 0)
  line L41 (845.1428, 0) -> (845.5908, 0)
  arc A20 (849.3618, 0) -> (845.5908, 0) centre (847.4763, -2.3335) ccw
  line L42 (849.3618, 0) -> (988, 0)
  line L43 (988, 0) -> (988, 602)
  line L44 (988, 602) -> (849.3618, 602)
  arc A21 (845.5908, 602) -> (849.3618, 602) centre (847.4763, 604.3335) ccw
  line L45 (845.5908, 602) -> (845.1428, 602)
  line L46 (845.1428, 602) -> (845.1428, 602.448)
  arc A22 (845.1428, 606.2189) -> (845.1428, 602.448) centre (847.4763, 604.3335) ccw
  line L47 (845.1428, 606.2189) -> (845.1428, 614)
  line L48 (845.1428, 614) -> (702.2857, 614)
  line L49 (702.2857, 614) -> (702.2857, 606.2189)
  arc A23 (702.2857, 602.448) -> (702.2857, 606.2189) centre (699.9523, 604.3335) ccw
  line L50 (702.2857, 602.448) -> (702.2857, 602)
  line L51 (702.2857, 602) -> (701.8377, 602)
  arc A24 (698.0668, 602) -> (701.8377, 602) centre (699.9523, 604.3335) ccw
  line L52 (698.0668, 602) -> (563.6475, 602)
  arc A25 (559.8765, 602) -> (563.6475, 602) centre (561.762, 604.3335) ccw
  line L53 (559.8765, 602) -> (559.4286, 602)
  line L54 (559.4286, 602) -> (559.4286, 602.448)
  arc A26 (559.4286, 606.2189) -> (559.4286, 602.448) centre (561.762, 604.3335) ccw
  line L55 (559.4286, 606.2189) -> (559.4286, 614)
  line L56 (559.4286, 614) -> (416.5714, 614)
  line L57 (416.5714, 614) -> (416.5714, 606.2189)
  arc A27 (416.5714, 602.448) -> (416.5714, 606.2189) centre (414.238, 604.3335) ccw
  line L58 (416.5714, 602.448) -> (416.5714, 602)
  line L59 (416.5714, 602) -> (416.1234, 602)
  arc A28 (412.3525, 602) -> (416.1234, 602) centre (414.238, 604.3335) ccw
  line L60 (412.3525, 602) -> (277.9332, 602)
  arc A29 (274.1623, 602) -> (277.9332, 602) centre (276.0477, 604.3335) ccw
  line L61 (274.1623, 602) -> (273.7143, 602)
  line L62 (273.7143, 602) -> (273.7143, 602.448)
  arc A30 (273.7143, 606.2189) -> (273.7143, 602.448) centre (276.0477, 604.3335) ccw
  line L63 (273.7143, 606.2189) -> (273.7143, 614)
  line L64 (273.7143, 614) -> (130.8571, 614)
  line L65 (130.8571, 614) -> (130.8571, 606.2189)
  arc A31 (130.8571, 602.448) -> (130.8571, 606.2189) centre (128.5237, 604.3335) ccw
  line L66 (130.8571, 602.448) -> (130.8571, 602)
  line L67 (130.8571, 602) -> (130.4092, 602)
  circle A32 centre (40, 301) radius 4
  circle A33 centre (390, 301) radius 4
  circle A34 centre (740, 301) radius 4
  point P0 (128.5237, 604.3335)
  point P1 (128.5237, -2.3335)
  point P2 (276.0477, -2.3335)
  point P3 (414.238, -2.3335)
  point P4 (847.4763, 604.3335)
  point P5 (414.238, 604.3335)
  point P6 (276.0477, 604.3335)
  point P7 (699.9523, 604.3335)
  point P8 (561.762, 604.3335)
  point P9 (561.762, -2.3335)
  point P10 (699.9523, -2.3335)
  point P11 (847.4763, -2.3335)
  point P12 (-2.3335, 240.7335)
  point P13 (-2.3335, 491.1335)
  point P14 (-2.3335, 361.2665)
  point P15 (-2.3335, 110.8665)
hole "Perçage4" at (-604.3335, 128.5237, 12) direction (0, 0, -1) diameter 6 depth 12 tip angle 180 bodies 12 in component "Component''''"
hole "Perçage5" at (2.3335, 128.5237, 12) at (2.3335, 276.0477, 12) at (2.3335, 414.238, 12) at (-604.3335, 847.4763, 12) at (-604.3335, 414.238, 12) at (-604.3335, 276.0477, 12) at (-604.3335, 699.9523, 12) at (-604.3335, 561.762, 12) at (2.3335, 561.762, 12) at (2.3335, 699.9523, 12) at (2.3335, 847.4763, 12) direction (0, 0, -1) diameter 6 depth 12 tip angle 180 bodies 12 in component "Component''''"
hole "Perçage6" at (-240.7335, -2.3335, 12) at (-491.1335, -2.3335, 12) at (-361.2665, -2.3335, 12) at (-110.8665, -2.3335, 12) direction (0, 0, -1) diameter 6 depth 12 tip angle 180 bodies 12 in component "Component''''"
sketch "Esquisse1 (7)" plane through (0, 0, -180) normal (0, 0, 1) x (0, 1, 0) in component "Component'''"
  line L0 (0, 0) -> (130.8571, 0)
  line L1 (130.8571, 0) -> (130.8571, -12)
  line L2 (130.8571, -12) -> (273.7143, -12)
  line L3 (273.7143, -12) -> (273.7143, 0)
  line L4 (273.7143, 0) -> (416.5714, 0)
  line L5 (416.5714, 0) -> (416.5714, -12)
  line L6 (416.5714, -12) -> (559.4286, -12)
  line L7 (559.4286, -12) -> (559.4286, 0)
  line L8 (559.4286, 0) -> (702.2857, 0)
  line L9 (702.2857, 0) -> (702.2857, -12)
  line L10 (702.2857, -12) -> (845.1428, -12)
  line L11 (845.1428, -12) -> (845.1428, 0)
  line L12 (845.1428, 0) -> (988, 0)
  line L13 (988, 0) -> (988, 602)
  line L14 (988, 602) -> (845.1428, 602)
  line L15 (845.1428, 602) -> (845.1428, 614)
  line L16 (845.1428, 614) -> (702.2857, 614)
  line L17 (702.2857, 614) -> (702.2857, 602)
  line L18 (702.2857, 602) -> (559.4286, 602)
  line L19 (559.4286, 602) -> (559.4286, 614)
  line L20 (559.4286, 614) -> (416.5714, 614)
  line L21 (416.5714, 614) -> (416.5714, 602)
  line L22 (416.5714, 602) -> (273.7143, 602)
  line L23 (273.7143, 602) -> (273.7143, 614)
  line L24 (273.7143, 614) -> (130.8571, 614)
  line L25 (130.8571, 614) -> (130.8571, 602)
  line L26 (130.8571, 602) -> (0, 602)
  line L27 (0, 602) -> (0, 488.8)
  line L28 (0, 488.8) -> (-12, 488.8)
  line L29 (-12, 488.8) -> (-12, 363.6)
  line L30 (-12, 363.6) -> (0, 363.6)
  line L31 (0, 363.6) -> (0, 238.4)
  line L32 (0, 238.4) -> (-12, 238.4)
  line L33 (-12, 238.4) -> (-12, 113.2)
  line L34 (-12, 113.2) -> (0, 113.2)
  line L35 (0, 113.2) -> (0, 0)
  point P0 (-2.3335, 491.1335)
  point P1 (-2.3335, 361.2665)
  point P2 (-2.3335, 240.7335)
  point P3 (-2.3335, 110.8665)
  point P4 (276.0477, 604.3335)
  point P5 (128.5237, 604.3335)
  point P6 (847.4763, 604.3335)
  point P7 (699.9523, 604.3335)
  point P8 (561.762, 604.3335)
  point P9 (414.238, 604.3335)
  point P10 (561.762, -2.3335)
  point P11 (414.238, -2.3335)
  point P12 (699.9523, -2.3335)
  point P13 (276.0477, -2.3335)
  point P14 (128.5237, -2.3335)
  point P15 (847.4763, -2.3335)
hole "Perçage1'''''" at (-491.1335, -2.3335, -180) at (-361.2665, -2.3335, -180) at (-240.7335, -2.3335, -180) at (-110.8665, -2.3335, -180) direction (0, 0, -1) diameter 6 depth 12 tip angle 180 bodies 11 in component "Component'''"
hole "Perçage2'''''" at (-604.3335, 699.9523, -180) at (2.3335, 699.9523, -180) direction (0, 0, -1) diameter 6 depth 12 tip angle 180 bodies 11 in component "Component'''"
hole "Perçage3'" at (-604.3335, 847.4763, -180) at (2.3335, 847.4763, -180) direction (0, 0, -1) diameter 6 depth 12 tip angle 180 bodies 11 in component "Component'''"
hole "Perçage4'" at (-604.3335, 276.0477, -180) at (2.3335, 276.0477, -180) direction (0, 0, -1) diameter 6 depth 12 tip angle 180 bodies 11 in component "Component'''"
hole "Perçage5'" at (-604.3335, 128.5237, -180) at (2.3335, 128.5237, -180) direction (0, 0, -1) diameter 6 depth 12 tip angle 180 bodies 11 in component "Component'''"
hole "Perçage6'" at (-604.3335, 561.762, -180) at (2.3335, 561.762, -180) direction (0, 0, -1) diameter 6 depth 12 tip angle 180 bodies 11 in component "Component'''"
hole "Perçage7" at (-604.3335, 414.238, -180) at (2.3335, 414.238, -180) direction (0, 0, -1) diameter 6 depth 12 tip angle 180 bodies 11 in component "Component'''"
component "Component" placed x (0, -1, 0) y (0, 0, 1) z (-1, 0, 0) at (-1211.3712, 12, 3005.5)
component "Component'" placed x (0, 0, -1) y (1, 0, 0) z (0, -1, 0) at (-513.4713, -593, 2748)
component "Component''" placed x (0, 1, 0) y (0, 0, -1) z (-1, 0, 0) at (-1211.2991, 614, 2842.0688)
component "Component'''" placed x (0, 0, -1) y (-1, 0, 0) z (0, 1, 0) at (-255.5, 192, 227.0686)
component "Component''''" placed x (-1, 0, 0) y (0, 0, 1) z (0, 1, 0) at (-1231.5, 0, 859.5688)
component "Component'''''" placed x (1, 0, 0) y (0, 1, 0) z (0, 0, 1) at (-53.1414, 12, 3961.5)
component "Component''''''" placed x (-1, 0, 0) y (0, 1, 0) z (0, 0, -1) at (-655.0692, 32, 1886.0688)
equation "d15 = ( 1000 / 7 ) * 1 mm"
equation "d23 = ( -1000 / 7 ) * 1 mm"
equation "d28 = ( 637 / 7 ) * 1 mm"
equation "d31 = ( -637 / 7 ) * 1 mm"
equation "d33 = ( -602 / 2 ) * 1 mm"
equation "d82 = ( 626 / 5 ) * 1 mm"
equation "d95 = -125.20 mm * 2"
